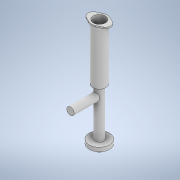
# Autodesk Inventor part: Syringe Lower
Saved by Autodesk Inventor 2022 (Build 260153000, 153)
## iProperties
Created: 2021-12-01
Part Number: Syringe Lower
Material: Generic
Document SubType Name: Modeling
Designer: efred
Density: 1 g/cm^3
Appearance: Default
Author: efred
Autodesk Inventor part; units mm, degrees
ref_plane "YZ Plane" through (0, 0, 0) normal (1, 0, 0) x (0, 1, 0)
ref_plane "XZ Plane" through (0, 0, 0) normal (0, 1, 0) x (-1, 0, 0)
ref_plane "XY Plane" through (0, 0, 0) normal (0, 0, 1) x (1, 0, 0)
sketch "Sketch1" plane through (0, 0, 0) normal (0, 1, 0) x (-1, 0, 0)
  circle A0 centre (0, 0) radius 10.65
  dimension "d0" = 21.3
  constraints: 1 centre point, 1 coincident
  measures "d0" diameter of A0
extrude "Extrusion1" add sketch "Sketch1" along normal blind 91
sketch "Sketch2" plane through (0, 91, 0) normal (0, 1, 0) x (1, 0, 0)
  circle A0 centre (0, 0) radius 9.9
  dimension "d3" = 19.8
  constraints: 1 centre point, 1 coincident
  measures "d3" diameter of A0
extrude "Extrusion2" cut sketch "Sketch2" against normal blind 90
sketch "Sketch3" plane through (0, 0, 0) normal (0, -1, 0) x (1, 0, 0)
  circle A0 centre (0, 0) radius 10.65 projected
  circle A1 centre (0, 0) radius 6.75
  dimension "d6" = 13.5
  constraints: 1 centre point, 1 coincident
  measures "d6" diameter of A1
extrude "Extrusion3" add sketch "Sketch3" along normal blind 77.8 contours A1
sketch "Sketch4" plane through (0, -77.8, 0) normal (0, -1, 0) x (1, 0, 0)
  circle A0 centre (0, 0) radius 6.75 projected
  circle A1 centre (0, 0) radius 16.6
  dimension "d9" = 33.2
  constraints: 1 centre point, 1 coincident
  measures "d9" diameter of A1
extrude "Extrusion4" add sketch "Sketch4" along normal blind 6.5 contours A0 | A1
sketch "Sketch5" plane through (0, -84.3, 0) normal (0, -1, 0) x (1, 0, 0)
  circle A0 centre (0, 0) radius 4.95
  dimension "d12" = 9.9
  constraints: 1 centre point, 1 coincident
  measures "d12" diameter of A0
extrude "Extrusion5" add sketch "Sketch5" along normal blind 8.8
sketch "Sketch6" plane through (0, 0, 0) normal (1, 0, 0) x (0, 1, 0)
  circle A0 centre (-15, 0) radius 6.1
  line L0 (0, -10.65) -> (0, 10.65) projected
  point P0 (0, 0)
  point P1 (0, 0)
  dimension "d15" = 15
  dimension "d16" = 12.2
  constraints: 1 centre point, 1 horizontal alignment, 1 midpoint
  measures "d15" distance from line of L0 A0.centre
  measures "d16" diameter of A0
extrude "Extrusion6" add sketch "Sketch6" along normal blind 47
sketch "Sketch7" plane through (0, 91, 0) normal (0, 1, 0) x (1, 0, 0)
  circle A0 centre (0, 0) radius 10.65 projected
  circle A1 centre (0, 0) radius 12.85
  arc A2 (13.7583, -7.5) -> (13.7583, 7.5) centre (10.0199, 0) ccw
  line L0 (13.7583, 7.5) -> (5.7324, 11.5005)
  line L1 (13.7583, -7.5) -> (5.7324, -11.5005)
  circle A3 centre (0, 0) radius 9.9 projected
  line L2 (0, 12.85) -> (0, -12.85) construction
  arc A4 (-13.7583, 7.5) -> (-13.7583, -7.5) centre (-10.0199, 0) ccw
  line L3 (-13.7583, 7.5) -> (-5.7324, 11.5005)
  line L4 (-13.7583, -7.5) -> (-5.7324, -11.5005)
  point P0 (9.9, 0)
  point P1 (18.4, 0)
  dimension "d19" = 25.7
  dimension "d22" = 8.5
  dimension "d23" = 15
  constraints: 10 end point, 9 point on circle, 5 symmetric about line, 4 horizontal alignment, 4 tangent, 3 centre point, 2 coincident, 1 midpoint, 1 vertical, 2 other
  measures "d19" diameter of A1
  measures "d22" distance of point (9.9, 0) point (18.4, 0)
  measures "d23" distance of L1.start L0.start
extrude "Extrusion7" add sketch "Sketch7" against normal blind 2.2 contours A1 | A1 L0 A2 L1 | A1 L4 A4 L3
pattern_circular "Circular Pattern1" count 2 over 90 about axis through (0, 0, 0) along (0, -1, 0) of "Extrusion6"
sketch "Sketch8" plane through (47, -15, 0) normal (1, 0, 0) x (0, 0, -1)
  circle A0 centre (0, 0) radius 6.1 projected
  point P0 (0, 15)
extrude "Extrusion8" cut sketch "Sketch8" against normal up to surface round surface about axis through (0, 0, 0) along (0, -1, 0) radius 6.75 far side no
body "Solid1"
